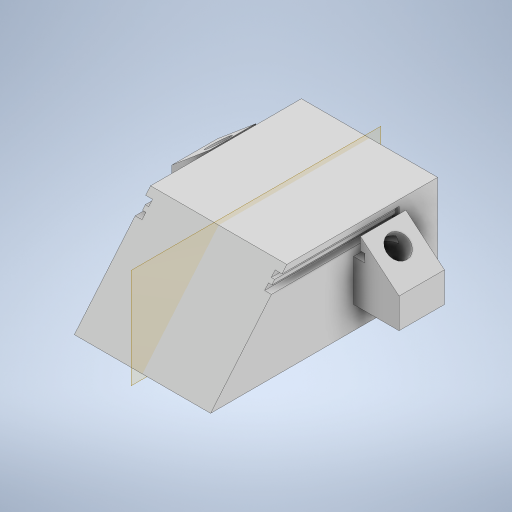
# Autodesk Inventor part: taslak2
Saved by Autodesk Inventor 2023 (Build 270158000, 158)
## iProperties
Created: 2023-03-22
Part Number: taslak2
Material: Generic
Document SubType Name: Modeling
Designer: Umut Yücesoy
Density: 1 g/cm^3
Appearance: Default
Author: Umut Yücesoy
Autodesk Inventor part; units mm, degrees
ref_plane "YZ Plane" through (0, 0, 0) normal (1, 0, 0) x (0, 1, 0)
ref_plane "XZ Plane" through (0, 0, 0) normal (0, 1, 0) x (-1, 0, 0)
ref_plane "XY Plane" through (0, 0, 0) normal (0, 0, 1) x (1, 0, 0)
sketch "Sketch1" plane through (0, 0, 0) normal (0, 1, 0) x (-1, 0, 0)
  line L0 (0, 0) -> (60, 0)
  line L1 (60, 0) -> (60, -100)
  line L2 (60, -100) -> (0, -100)
  line L3 (0, -100) -> (0, 0)
  dimension "d0" = 100
  dimension "d1" = 60
  constraints: 8 end point, 2 parallel, 1 horizontal, 1 perpendicular
  measures "d0" distance of L0.end L1.end
  measures "d1" distance of L1.end L2.end
extrude "Extrusion1" add sketch "Sketch1" along normal blind 40
sketch "Sketch2" plane through (0, 0, 0) normal (1, 0, 0) x (0, 0, -1)
  line L0 (0, 0) -> (37.6485, 44.8677)
  line L1 (0, 0) -> (58.5706, 0) construction
  line L2 (100, 40) -> (0, 40) projected
  line L3 (0, 40) -> (0, 0)
  point P0 (33.564, 40)
  dimension "d4" = 50
  constraints: 6 end point, 1 equal length, 1 horizontal, 1 perpendicular
  measures "d4" angle of L1 L0
extrude "Extrusion2" cut sketch "Sketch2" against normal blind 70
sketch "Sketch3" plane through (0, 0, -100) normal (1, 0, 0) x (0, 0, -1)
  line L0 (0, 0) -> (-17, 0)
  line L1 (-100, 0) -> (0, 0) projected
  line L2 (0, 40) -> (-66.436, 40) projected
  line L3 (-17, 40) -> (-37, 40)
  line L4 (-37, 40) -> (-37, 10)
  line L5 (-37, 10) -> (-17, 10)
  line L6 (-17, 10) -> (-17, 40)
  dimension "d7" = 17
  dimension "d8" = 20
  dimension "d9" = 30
  constraints: 10 end point, 3 point on line, 1 parallel, 1 perpendicular, 1 vertical
  measures "d7" distance of L0.start L0.end
  measures "d8" distance of L3.start L3.end
  measures "d9" distance of L3.end L4.end
extrude "Extrusion3" add sketch "Sketch3" along normal blind 20
sketch "Sketch4" plane through (0, 10, -63) normal (0, 0, 1) x (1, 0, 0)
  line L0 (0, 30) -> (-60, 30) projected
  line L1 (0, 30) -> (29.4147, 5.3181)
  line L2 (0, 30) -> (38.3982, 30) construction
  line L3 (0, 30) -> (20, 30) projected
  line L4 (0, 30) -> (20, 30)
  line L5 (20, 30) -> (20, 13.218)
  line L6 (20, 0) -> (20, 30) projected
  point P0 (0, -10)
  dimension "d12" = 40
  constraints: 8 end point, 4 point on line, 1 collinear, 1 equal length, 1 horizontal
  measures "d12" angle of L1 L2
extrude "Extrusion4" cut sketch "Sketch4" against normal blind 61.75
ref_plane "Work Plane1" through (-30, 0, -100) normal (1, 0, 0) x (0, 0, -1)
mirror "Mirror1" about plane through (-30, 0, -100) normal (1, 0, 0) of "Extrusion3", "Extrusion4"
sketch "Sketch5" plane through (0, 40, -63) normal (0.6428, 0.766, 0) x (0.766, -0.6428, 0)
  circle A0 centre (12.5, 10) radius 5
  point P0 (25.7115, -63)
  dimension "d16" = 10
  constraints: 1 centre point
  measures "d16" diameter of A0
extrude "Extrusion5" cut sketch "Sketch5" against normal blind 27
mirror "Mirror2" about plane through (-30, 0, -100) normal (1, 0, 0) of "Extrusion5"
sketch "Sketch6" plane through (20, 10, -83) normal (0, 0, -1) x (-1, 0, 0)
  line L0 (14.2547, 25.1791) -> (31.6099, 4.4959) projected
  line L1 (6.5942, 18.7512) -> (23.9495, -1.932) projected
  line L2 (20, 30) -> (20, 18.3321)
  line L3 (20, 30) -> (20, 0) projected
  line L4 (20, 18.3321) -> (17, 18.3321)
  line L5 (17, 18.3321) -> (17, 27.4827)
  line L6 (17, 27.4827) -> (20, 30)
  line L7 (20, 23.9074) -> (20, 30)
  line L8 (20, 23.9074) -> (20, 30)
  point P0 (20, -10)
  dimension "d19" = 3
  constraints: 12 end point, 3 point on line, 2 collinear, 1 horizontal, 1 perpendicular
  measures "d19" distance of L2.end L4.end
extrude "Extrusion6" cut sketch "Sketch6" against normal blind 81
mirror "Mirror3" about plane through (-30, 0, -100) normal (1, 0, 0) of "Extrusion6"
sketch "Sketch7" plane through (0, 0, -100) normal (0, 0, -1) x (-1, 0, 0)
  line L0 (-3, 28.3321) -> (0, 28.3321) projected
  line L1 (-0.0001, 31.9514) -> (2.9999, 31.9514)
  line L2 (2.9999, 31.9514) -> (2.9999, 33.9514)
  line L3 (1.4999, 33.9514) -> (2.9999, 33.9514)
  line L4 (1.4999, 33.9514) -> (1.4999, 35.4514)
  line L5 (1.4999, 35.4514) -> (2.9999, 35.4514)
  line L6 (2.9999, 35.4514) -> (2.9999, 37.4514)
  line L7 (2.9999, 37.4514) -> (-0.0001, 37.4514)
  line L8 (0, 0) -> (0, 40) projected
  line L9 (0, 37.4515) -> (0, 40)
  line L10 (-0.0001, 37.4514) -> (-0.0001, 31.9514)
  point P0 (0, 37.4514)
  point P1 (0, 31.9514)
  dimension "d23" = 2
  dimension "d24" = 1.5
  dimension "d25" = 2
  dimension "d26" = 1.5
  dimension "d27" = 5.5
  dimension "d28" = 3
  constraints: 18 end point, 5 perpendicular, 3 point on line, 1 collinear, 1 horizontal, 1 parallel
  measures "d23" distance of L1.end L2.end
  measures "d24" distance of L3.start L4.end
  measures "d25" distance of L5.end L6.end
  measures "d26" distance of L3.start L2.end
  measures "d27" distance of L1.start L7.end
  measures "d28" distance of L1.start L1.end
extrude "Extrusion7" cut sketch "Sketch7" against normal blind 92.75
sketch "Sketch8" plane through (0, 0, -100) normal (0, 0, -1) x (-1, 0, 0)
  line L0 (2.9999, 37.4514) -> (0, 37.4514) projected
  line L1 (2.9999, 37.4514) -> (0, 37.4514)
  line L2 (0, 31.9514) -> (2.9999, 31.9514) projected
  line L3 (0, 37.4514) -> (0, 31.9514)
  line L4 (0, 31.9514) -> (2.9999, 31.9514)
  line L5 (2.9999, 31.9514) -> (2.9999, 33.9514) projected
  line L6 (2.9999, 31.9514) -> (2.9999, 33.9514)
  line L7 (2.9999, 33.9514) -> (1.4999, 33.9514)
  line L8 (1.4999, 35.4514) -> (1.4999, 33.9514) projected
  line L9 (1.4999, 33.9514) -> (1.4999, 35.4514)
  line L10 (1.4999, 35.4514) -> (2.9999, 35.4514)
  line L11 (2.9999, 35.4514) -> (2.9999, 37.4514)
  point P0 (0, 0)
  constraints: 16 end point, 6 perpendicular, 1 collinear, 1 horizontal, 1 point on line
extrude "Extrusion8" add sketch "Sketch8" against normal blind 17
sketch "Sketch9" plane through (20, 10, -83) normal (0, 0, -1) x (-1, 0, 0)
  line L0 (17, 18.3321) -> (20, 18.3321) projected
  line L1 (17, 18.3321) -> (17, 21.9514)
  line L2 (17, 18.3321) -> (17, 27.4827) projected
  line L3 (17, 21.9514) -> (15, 21.9514)
  line L4 (15, 21.9514) -> (15, 18.3321)
  line L5 (15, 18.3321) -> (17, 18.3321)
  point P0 (20, -10)
  point P1 (20, 21.9514)
  dimension "d33" = 2
  dimension "d34" = 3.6194
  constraints: 8 end point, 3 perpendicular, 1 point on line
  measures "d33" distance of L1.end L3.end
  measures "d34" distance of L3.end L4.end
extrude "Extrusion9" cut sketch "Sketch9" against normal blind 69.75
mirror "Mirror4" about plane through (-30, 0, -100) normal (1, 0, 0) of "Extrusion7", "Extrusion9"
sketch "Sketch10" plane through (0, 0, -100) normal (0, 0, -1) x (-1, 0, 0)
  line L0 (60, 0) -> (60, 31.9514) projected
  line L1 (57.0001, 31.9514) -> (60, 31.9514) projected
  line L2 (60, 31.9514) -> (57.0001, 31.9514)
  line L3 (57.0001, 33.9514) -> (57.0001, 31.9514) projected
  line L4 (57.0001, 31.9514) -> (57.0001, 33.9514)
  line L5 (57.0001, 33.9514) -> (58.5001, 33.9514)
  line L6 (58.5001, 35.4514) -> (58.5001, 33.9514) projected
  line L7 (58.5001, 33.9514) -> (58.5001, 35.4514)
  line L8 (57.0001, 35.4514) -> (58.5001, 35.4514) projected
  line L9 (58.5001, 35.4514) -> (57.0001, 35.4514)
  line L10 (57.0001, 37.4514) -> (57.0001, 35.4514) projected
  line L11 (57.0001, 35.4514) -> (57.0001, 37.4514)
  line L12 (60, 37.4514) -> (57.0001, 37.4514) projected
  line L13 (57.0001, 37.4514) -> (60, 37.4514)
  line L14 (60, 37.4514) -> (60, 31.9514)
  point P0 (0, 0)
  constraints: 16 end point, 4 collinear, 4 perpendicular
extrude "Extrusion10" add sketch "Sketch10" against normal blind 17
sketch "Sketch11" plane through (0, 0, -100) normal (0, 0, -1) x (-1, 0, 0)
  point P0 (0, 0)
body "Solid1"
